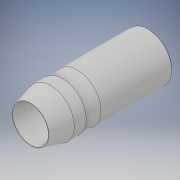
# Autodesk Inventor part: douille
Saved by Autodesk Inventor 2019 (Build 230136000, 136)
## iProperties
Created: 2019-03-19
Part Number: douille
Material: Générique
Document SubType Name: Modeling
Designer: theor
Density: 1 g/cm^3
Appearance: Par défaut
Author: theor
Autodesk Inventor part; units mm, degrees
ref_plane "YZ Plane" through (0, 0, 0) normal (1, 0, 0) x (0, 1, 0)
ref_plane "XZ Plane" through (0, 0, 0) normal (0, 1, 0) x (-1, 0, 0)
ref_plane "XY Plane" through (0, 0, 0) normal (0, 0, 1) x (1, 0, 0)
sketch "Esquisse1" plane through (0, 0, 0) normal (1, 0, 0) x (0, 1, 0)
  line L0 (0, 0) -> (0, -10.1548)
  line L1 (6, 0) -> (6, -30)
  line L2 (6, 0) -> (6.2, 0)
  line L3 (6.2, 0) -> (8, -6.7177)
  line L4 (8, -6.7177) -> (8, -10.7177)
  line L5 (7, -40) -> (8, -40)
  line L6 (7, -40) -> (6, -30)
  line L7 (8, -10.7177) -> (7, -10.7177)
  line L8 (7, -10.7177) -> (8, -15.7177)
  line L9 (8, -15.7177) -> (8, -40)
  dimension "d4" = 12
  dimension "d5" = 0.2
  dimension "d6" = 40
  dimension "d10" = 165
  dimension "d11" = 16
  dimension "d15" = 10
  dimension "d16" = 14
  dimension "d17" = 5
  dimension "d18" = 1
  dimension "d19" = 4
  constraints: 20 end point, 4 vertical, 3 horizontal, 1 collinear, 1 horizontal alignment
  measures "d4" diameter of L1 L0
  measures "d5" distance of L1.start L2.end
  measures "d6" distance from line of L5 L2.end
  measures "d10" angle of L3 L4
  measures "d11" diameter of L4 L0
  measures "d15" vertical distance of L5.start L1.end
  measures "d16" diameter of L5.start L0
  measures "d17" distance from line of L8.end L7
  measures "d18" distance of L4.end L7.end
  measures "d19" distance of L3.end L4.end
revolve "Révolution1" add sketch "Esquisse1" angle 360 about axis through (0, 0, 0) along (0, 0, -1)
chamfer "Chanfrein1" distance 0.5 angle 45 1 edges at (0, -8, -40)
